Autodesk Inventor part; units mm, degrees
(part 2 of 2)
sketch "Sketch10" plane through (12.7, -57.9553, 48.26) normal (1, 0, 0) x (0, 0, -1)
  line L0 (238.76, 169.0803) -> (-142.24, 169.0803) projected
  circle A0 centre (-74.422, 78.5928) radius 3.175 projected
  circle A1 centre (-74.422, 103.9928) radius 3.175 projected
  circle A2 centre (48.26, 57.9553) radius 3.175 projected
  circle A3 centre (-48.26, 57.9553) radius 3.175 projected
  circle A4 centre (144.78, 57.9553) radius 3.175 projected
  circle A5 centre (-205.74, 124.6303) radius 12.7 projected
  circle A6 centre (302.26, 124.6303) radius 12.7 projected
  line L1 (-205.74, 124.6303) -> (302.26, 124.6303) construction
  line L2 (48.26, 124.6303) -> (48.26, 202.3568) construction
  circle A7 centre (-133.9387, 147.2642) radius 2.413 projected
  circle A8 centre (-131.9736, 159.9642) radius 2.413 projected
  circle A9 centre (230.4587, 147.2642) radius 2.413
  circle A10 centre (228.4936, 159.9642) radius 2.413
  line L3 (238.76, 169.0803) -> (239.9837, 147.2642)
  arc A11 (230.4587, 137.7392) -> (239.9837, 147.2642) centre (230.4587, 147.2642) ccw
  spline S0 degree 4 poles (180.4444, 121.0575) (193.8696, 130.2235) (215.0032, 150.2263) (220.4765, 137.7392) (230.4587, 137.7392) knots 0 0 0 0 0 1 1 1 1 1
  circle A12 centre (81.2991, 80.8647) radius 2.0193 projected
  line L4 (-142.24, 169.0803) -> (-142.24, 124.4818) projected
  arc A13 (-110.574, 77.2765) -> (-142.24, 124.4818) centre (-128.865, 99.2303) ccw projected
  line L5 (-110.574, 77.2765) -> (-54.3105, 46.7892) projected
  arc A14 (-54.3105, 46.7892) -> (-42.2095, 46.7892) centre (-48.26, 57.9553) ccw projected
  line L6 (-42.2095, 46.7892) -> (-7.5631, 65.5629) projected
  arc A15 (7.5631, 65.5629) -> (-7.5631, 65.5629) centre (0, 51.6053) ccw projected
  line L7 (7.5631, 65.5629) -> (42.2095, 46.7892) projected
  arc A16 (42.2095, 46.7892) -> (54.3105, 46.7892) centre (48.26, 57.9553) ccw projected
  line L8 (54.3105, 46.7892) -> (88.9569, 65.5629) projected
  arc A17 (104.0831, 65.5629) -> (88.9569, 65.5629) centre (96.52, 51.6053) ccw projected
  line L9 (104.0831, 65.5629) -> (138.7295, 46.7892) projected
  arc A18 (138.7295, 46.7892) -> (150.8305, 46.7892) centre (144.78, 57.9553) ccw projected
  line L10 (150.8305, 46.7892) -> (207.094, 77.2765) projected
  arc A19 (238.76, 124.4818) -> (207.094, 77.2765) centre (225.385, 99.2303) ccw projected
  line L11 (238.76, 124.4818) -> (238.76, 169.0803) projected
  point P0 (215.721, 140.529)
  dimension "d83" = 254
  constraints: 6 end point, 3 centre point, 2 point on circle, 2 symmetric about line, 1 horizontal, 1 midpoint, 1 vertical, 6 other
  measures "d83" distance from line of L2 L1.start
extrude "Extrusion12" [suppressed]
sketch "Sketch11" plane through (12.7, -57.9553, 48.26) normal (1, 0, 0) x (0, 0, -1)
  circle A0 centre (228.4936, 159.9642) radius 2.413 projected
  circle A1 centre (228.4936, 159.9642) radius 2.413
  point P0 (48.26, 57.9553)
  constraints: 1 centre point, 1 coincident, 1 concentric
extrude "Extrusion13" [suppressed]
sketch "Sketch12" plane through (12.7, -57.9553, 48.26) normal (1, 0, 0) x (0, 0, -1)
  circle A0 centre (224.987, 100.468) radius 6.35 construction
  circle A1 centre (173.2834, 131.5461) radius 6.35 projected
  circle A2 centre (-97.79, 143.6803) radius 7.9375 projected
  circle A3 centre (-47.752, 156.3803) radius 2.0193
  line L0 (238.76, 169.0803) -> (-142.24, 169.0803) projected
  line L1 (44.2912, 144.6069) -> (44.2912, 72.043) projected
  line L2 (97.5225, 158.7615) -> (97.5225, 118.5822) projected
  circle A4 centre (-22.352, 156.3803) radius 2.0193
  circle A5 centre (-47.752, 130.9803) radius 2.0193
  circle A6 centre (-22.352, 130.9803) radius 2.0193
  circle A7 centre (66.04, 105.5803) radius 2.0193
  circle A8 centre (91.44, 105.5803) radius 2.0193
  circle A9 centre (66.04, 80.1803) radius 2.0193
  circle A10 centre (91.44, 80.1803) radius 2.0193
  circle A11 centre (-74.422, 103.9928) radius 3.175 projected
  circle A12 centre (-74.422, 78.5928) radius 3.175 projected
  circle A13 centre (140.335, 92.8803) radius 7.9375 projected
  circle A14 centre (144.78, 57.9553) radius 3.175 projected
  circle A15 centre (230.4587, 147.2642) radius 2.413 projected
  circle A16 centre (176.53, 89.5304) radius 3.175
  circle A17 centre (212.5643, 140.4513) radius 3.175
  circle A18 centre (173.2834, 131.5461) radius 29.845 construction
  circle A19 centre (140.335, 92.8803) radius 23.495 construction
  circle A20 centre (224.987, 100.468) radius 33.02 construction
  line L3 (144.78, 57.9553) -> (176.53, 89.5304) construction
  line L4 (176.53, 89.5304) -> (140.335, 92.8803) construction
  line L5 (176.53, 89.5304) -> (173.2834, 131.5461) construction
  line L6 (176.53, 89.5304) -> (212.5643, 140.4513) construction
  line L7 (212.5643, 140.4513) -> (230.4587, 147.2642) construction
  line L8 (212.5643, 140.4513) -> (173.2834, 131.5461) construction
  circle A21 centre (224.987, 100.468) radius 23.8125 construction
  circle A22 centre (176.53, 89.5304) radius 6.35 construction
  circle A23 centre (212.5643, 140.4513) radius 6.35 construction
  point P0 (48.26, 57.9553)
  dimension "d88" = 12.7
  dimension "d89" = 31.078
  dimension "d90" = 51.7036
  dimension "d94" = 4.0386
  dimension "d97" = 25.4
  dimension "d100" = 25.4
  dimension "d103" = 4.0386
  dimension "d106" = 25.4
  dimension "d109" = 25.4
  dimension "d112" = 50.038
  dimension "d113" = 12.7
  dimension "d114" = 48.895
  dimension "d115" = 12.7
  dimension "d116" = 6.35
  dimension "d117" = 6.35
  dimension "d118" = 59.69
  dimension "d119" = 46.99
  dimension "d120" = 66.04
  dimension "d121" = 47.625
  dimension "d122" = 31.75
  dimension "d124" = 12.7
  dimension "d125" = 12.7
  constraints: 17 centre point, 12 end point, 6 coincident, 2 horizontal, 2 vertical, 12 other
  measures "d88" diameter of A0
  measures "d89" vertical distance of A0.centre A1.centre
  measures "d90" horizontal distance of A0.centre A1.centre
  measures "d94" diameter of A3
  measures "d97" distance of A3.centre A4.centre
  measures "d100" distance of A3.centre A5.centre
  measures "d103" diameter of A7
  measures "d106" distance of A7.centre A8.centre
  measures "d109" distance of A7.centre A9.centre
  measures "d112" horizontal distance of A5.centre A2.centre
  measures "d113" vertical distance of A5.centre A2.centre
  measures "d114" horizontal distance of A13.centre A10.centre
  measures "d115" vertical distance of A13.centre A10.centre
  measures "d116" diameter of A16
  measures "d117" diameter of A17
  measures "d118" diameter of A18
  measures "d119" diameter of A19
  measures "d120" diameter of A20
  measures "d121" diameter of A21
  measures "d122" horizontal distance of L3.end L3.start
  measures "d124" diameter of A22
  measures "d125" diameter of A23
fillet "Fillet4" [suppressed]
fillet "Fillet5" [suppressed]
sketch "Sketch13" plane through (12.7, 0, 0) normal (1, 0, 0) x (0, 0, -1)
  arc A0 (-155.8742, 22.1717) -> (-155.0257, 17.2576) centre (-153.513, 20.0491) ccw projected
  line L0 (-155.0257, 17.2576) -> (-102.5705, -11.1661) projected
  arc A1 (-102.5705, -11.1661) -> (-90.4695, -11.1661) centre (-96.52, 0) ccw projected
  line L1 (-90.4695, -11.1661) -> (-55.8231, 7.6076) projected
  arc A2 (-40.6969, 7.6076) -> (-55.8231, 7.6076) centre (-48.26, -6.35) ccw projected
  line L2 (-40.6969, 7.6076) -> (-6.0505, -11.1661) projected
  arc A3 (-6.0505, -11.1661) -> (6.0505, -11.1661) centre (0, 0) ccw projected
  line L3 (6.0505, -11.1661) -> (40.6969, 7.6076) projected
  arc A4 (55.8231, 7.6076) -> (40.6969, 7.6076) centre (48.26, -6.35) ccw projected
  line L4 (55.8231, 7.6076) -> (90.4695, -11.1661) projected
  arc A5 (90.4695, -11.1661) -> (102.5705, -11.1661) centre (96.52, 0) ccw projected
  line L5 (102.5705, -11.1661) -> (155.0257, 17.2576) projected
  arc A6 (155.0257, 17.2576) -> (155.8742, 22.1717) centre (153.513, 20.0491) ccw projected
  arc A7 (186.305, 68.3353) -> (155.8742, 22.1717) centre (177.125, 41.275) ccw projected
  arc A8 (186.305, 68.3353) -> (190.5, 71.342) centre (187.325, 71.342) ccw projected
  line L6 (190.5, 71.342) -> (190.5, 111.125) projected
  line L7 (190.5, 111.125) -> (-190.5, 111.125) projected
  line L8 (-190.5, 111.125) -> (-190.5, 71.342) projected
  arc A9 (-190.5, 71.342) -> (-186.305, 68.3353) centre (-187.325, 71.342) ccw projected
  arc A10 (-155.8742, 22.1717) -> (-186.305, 68.3353) centre (-177.125, 41.275) ccw projected
  circle A11 centre (-79.2324, 71.4375) radius 3.175 projected
  circle A12 centre (88.2841, 92.075) radius 3.175 projected
  circle A13 centre (182.1987, 89.3089) radius 2.413 projected
  circle A14 centre (-182.1987, 89.3089) radius 2.413 projected
  circle A15 centre (-107.3629, 85.725) radius 11 projected
  circle A16 centre (33.0391, 22.9094) radius 2.0193 projected
  circle A17 centre (-31.9249, 73.9625) radius 2.0193 projected
  circle A18 centre (-31.9249, 99.3625) radius 2.0193 projected
  circle A19 centre (33.0391, 48.3094) radius 2.0193 projected
  circle A20 centre (-57.3249, 99.3625) radius 2.0193 projected
  circle A21 centre (-122.682, 46.0375) radius 3.175 projected
  circle A22 centre (96.52, 0) radius 3.175 projected
  circle A23 centre (0, 0) radius 3.175 projected
  circle A24 centre (-96.52, 0) radius 3.175 projected
  circle A25 centre (-57.3249, 73.9625) radius 2.0193 projected
  circle A26 centre (58.4391, 48.3094) radius 2.0193 projected
  circle A27 centre (58.4391, 22.9094) radius 2.0193 projected
  circle A28 centre (-180.2336, 102.0089) radius 2.413 projected
  circle A29 centre (180.2336, 102.0089) radius 2.413 projected
  circle A30 centre (88.2841, 66.675) radius 3.175 projected
  circle A31 centre (-79.2324, 103.1875) radius 3.175 projected
  circle A32 centre (132.7341, 17.4625) radius 3.175 projected
  circle A33 centre (-147.5038, 79.375) radius 14.2875 projected
  circle A34 centre (-122.682, 20.6375) radius 3.175 projected
  line L9 (-187.325, 107.95) -> (187.325, 107.95)
  line L10 (187.325, 107.95) -> (187.325, 71.342)
  arc A35 (187.325, 71.342) -> (153.513, 20.0491) centre (177.125, 41.275) ccw
  line L11 (153.513, 20.0491) -> (101.0579, -8.3746)
  arc A36 (91.9821, -8.3746) -> (101.0579, -8.3746) centre (96.52, 0) ccw
  line L12 (91.9821, -8.3746) -> (57.3358, 10.3991)
  arc A37 (57.3358, 10.3991) -> (39.1842, 10.3991) centre (48.26, -6.35) ccw
  line L13 (39.1842, 10.3991) -> (4.5379, -8.3746)
  arc A38 (-4.5379, -8.3746) -> (4.5379, -8.3746) centre (0, 0) ccw
  line L14 (-4.5379, -8.3746) -> (-39.1842, 10.3991)
  arc A39 (-39.1842, 10.3991) -> (-57.3358, 10.3991) centre (-48.26, -6.35) ccw
  line L15 (-57.3358, 10.3991) -> (-91.9821, -8.3746)
  arc A40 (-101.0579, -8.3746) -> (-91.9821, -8.3746) centre (-96.52, 0) ccw
  line L16 (-101.0579, -8.3746) -> (-153.513, 20.0491)
  arc A41 (-153.513, 20.0491) -> (-187.325, 71.342) centre (-177.125, 41.275) ccw
  line L17 (-187.325, 71.342) -> (-187.325, 107.95)
  circle A42 centre (-147.5038, 79.375) radius 17.4625
  circle A43 centre (-107.3629, 85.725) radius 14.175
  circle A44 centre (-79.2324, 103.1875) radius 6.35
  circle A45 centre (-122.682, 46.0375) radius 6.35
  circle A46 centre (-122.682, 20.6375) radius 6.35
  circle A47 centre (-79.2324, 71.4375) radius 6.35
  circle A48 centre (88.2841, 66.675) radius 6.35
  circle A49 centre (88.2841, 92.075) radius 6.35
  circle A50 centre (132.7341, 17.4625) radius 6.35
  circle A51 centre (-57.3249, 99.3625) radius 5.1943
  circle A52 centre (-31.9249, 99.3625) radius 5.1943
  circle A53 centre (-57.3249, 73.9625) radius 5.1943
  circle A54 centre (-31.9249, 73.9625) radius 5.1943
  circle A55 centre (33.0391, 48.3094) radius 5.1943
  circle A56 centre (58.4391, 48.3094) radius 5.1943
  circle A57 centre (33.0391, 22.9094) radius 5.1943
  circle A58 centre (58.4391, 22.9094) radius 5.1943
  circle A59 centre (180.2336, 102.0089) radius 5.588
  circle A60 centre (182.1987, 89.3089) radius 5.588
  circle A61 centre (96.52, 0) radius 6.35
  circle A62 centre (0, 0) radius 6.35
  circle A63 centre (-96.52, 0) radius 6.35
  line L18 (-147.5038, 79.375) -> (-107.3629, 85.725) construction
  line L19 (-107.3629, 85.725) -> (-79.2324, 103.1875) construction
  line L20 (-79.2324, 103.1875) -> (-57.3249, 99.3625) construction
  line L21 (-57.3249, 99.3625) -> (-31.9249, 99.3625) construction
  line L22 (-31.9249, 99.3625) -> (88.2841, 92.075) construction
  line L23 (88.2841, 92.075) -> (135.2431, 65.2528) construction
  line L24 (108.4771, 34.6719) -> (132.7341, 17.4625) construction
  line L25 (132.7341, 17.4625) -> (96.52, 0) construction
  line L26 (96.52, 0) -> (58.4391, 22.9094) construction
  line L27 (58.4391, 22.9094) -> (33.0391, 48.3094) construction
  line L28 (33.0391, 48.3094) -> (-31.9249, 73.9625) construction
  line L29 (-31.9249, 73.9625) -> (-57.3249, 99.3625) construction
  line L30 (-147.5038, 79.375) -> (-122.682, 46.0375) construction
  line L31 (-122.682, 46.0375) -> (-122.682, 20.6375) construction
  line L32 (-122.682, 20.6375) -> (-96.52, 0) construction
  line L33 (-96.52, 0) -> (-79.2324, 71.4375) construction
  line L34 (-79.2324, 71.4375) -> (-57.3249, 73.9625) construction
  line L35 (-57.3249, 73.9625) -> (-31.9249, 73.9625) construction
  line L36 (-31.9249, 73.9625) -> (0, 0) construction
  line L37 (0, 0) -> (33.0391, 22.9094) construction
  line L38 (33.0391, 22.9094) -> (33.0391, 48.3094) construction
  line L39 (-107.3629, 85.725) -> (-79.2324, 71.4375) construction
  line L40 (-31.9249, 99.3625) -> (-31.9249, 73.9625) construction
  line L41 (-57.3249, 99.3625) -> (-57.3249, 73.9625) construction
  line L42 (33.0391, 48.3094) -> (58.4391, 48.3094) construction
  line L43 (58.4391, 48.3094) -> (58.4391, 22.9094) construction
  line L44 (33.0391, 22.9094) -> (58.4391, 22.9094) construction
  line L45 (108.4771, 34.6719) -> (58.4391, 22.9094) construction
  line L46 (108.4771, 34.6719) -> (58.4391, 48.3094) construction
  line L47 (108.4771, 34.6719) -> (88.2841, 66.675) construction
  line L48 (88.2841, 66.675) -> (135.2431, 65.2528) construction
  line L49 (88.2841, 66.675) -> (88.2841, 92.075) construction
  line L50 (108.4771, 34.6719) -> (135.2431, 65.2528) construction
  line L51 (135.2431, 65.2528) -> (182.1987, 89.3089) construction
  line L52 (135.2431, 65.2528) -> (180.2336, 102.0089) construction
  line L53 (88.2841, 92.075) -> (180.2336, 102.0089) construction
  line L54 (-180.2336, 102.0089) -> (-147.5038, 79.375) construction
  line L55 (-182.1987, 89.3089) -> (-147.5038, 79.375) construction
  circle A64 centre (135.2431, 65.2528) radius 14.2875 projected
  circle A65 centre (135.2431, 65.2528) radius 17.4625
  circle A66 centre (-180.2336, 102.0089) radius 5.588
  circle A67 centre (-182.1987, 89.3089) radius 5.588
  circle A68 centre (108.4771, 34.6719) radius 11 projected
  line L56 (132.7341, 17.4625) -> (135.2431, 65.2528) construction
  line L57 (58.4391, 48.3094) -> (88.2841, 66.675) construction
  line L58 (58.4391, 48.3094) -> (88.2841, 92.075) construction
  line L59 (33.0391, 48.3094) -> (-31.9249, 99.3625) construction
  line L60 (33.0391, 48.3094) -> (36.2167, 95.2315) construction
  line L61 (58.4391, 48.3094) -> (36.2167, 95.2315) construction
  line L62 (-57.3249, 73.9625) -> (-48.26, 12.7) construction
  line L63 (-122.682, 46.0375) -> (-79.2324, 71.4375) construction
  dimension "d300" = 3.175
  dimension "d301" = 3.175
  dimension "d302" = 3.175
  dimension "d303" = 3.175
  dimension "d304" = 3.175
  dimension "d307" = 3.175
  dimension "d308" = 3.175
  dimension "d309" = 3.175
  constraints: 110 end point, 32 centre point, 17 equal radius, 15 point on circle, 3 perpendicular, 2 coincident, 2 horizontal, 2 parallel, 1 point on line, 1 vertical, 15 other
  measures "d300" distance between parallel lines of L7 L9
  measures "d301" radial gap between concentric circles of A33 A42
  measures "d302" radial gap between concentric circles of A15 A43
  measures "d303" radial gap between concentric circles of A31 A44
  measures "d304" radial gap between concentric circles of A20 A51
  measures "d307" radial gap between concentric circles of A29 A59
  measures "d308" radial gap between concentric circles of A13 A60
  measures "d309" radial gap between concentric circles of A22 A61
sketch "Sketch14" plane through (12.7, 0, 0) normal (1, 0, 0) x (0, 0, -1)
  circle A0 centre (-147.5038, 79.375) radius 14.2875 projected
  circle A1 centre (-107.3629, 85.725) radius 11 projected
  circle A2 centre (108.4771, 34.6719) radius 11 projected
  circle A3 centre (135.2431, 65.2528) radius 14.2875 projected
  circle A4 centre (-147.5038, 79.375) radius 6.35
  circle A5 centre (-107.3629, 85.725) radius 6.35
  circle A6 centre (108.4771, 34.6719) radius 6.35
  circle A7 centre (135.2431, 65.2528) radius 6.35
  point P0 (0, 0)
  dimension "d327" = 12.7
  dimension "d328" = 12.7
  dimension "d329" = 12.7
  dimension "d330" = 12.7
  constraints: 4 centre point, 4 coincident
  measures "d327" diameter of A4
  measures "d328" diameter of A5
  measures "d329" diameter of A6
  measures "d330" diameter of A7
extrude "Extrusion14" [suppressed]
extrude "Extrusion15" [suppressed]
sketch "Sketch17" plane through (0, 0, 0) normal (1, 0, 0) x (0, 1, 0)
  circle A0 centre (80.3177, 148.0067) radius 2.54
  circle A1 centre (41.275, 177.125) radius 2.54
  circle A2 centre (46.0375, 122.682) radius 3.175 projected
  circle A3 centre (20.6375, 122.682) radius 3.175 projected
  circle A4 centre (80.3177, 148.0067) radius 7.62
  circle A5 centre (41.275, 177.125) radius 7.62
  line L0 (34.1796, 179.9035) -> (12.9508, 125.692)
  line L1 (45.8306, 183.2333) -> (84.8733, 154.115)
  line L2 (51.041, 116.1162) -> (84.9363, 141.946)
  line L3 (20.6375, 114.427) -> (46.0375, 114.427)
  circle A6 centre (46.0375, 122.682) radius 8.255
  circle A7 centre (20.6375, 122.682) radius 8.255
  point P0 (0, 0)
  dimension "d349" = 5.08
  dimension "d350" = 5.08
  dimension "d351" = 5.08
  dimension "d352" = 5.08
  dimension "d356" = 5.08
  dimension "d357" = 5.08
  constraints: 8 end point, 4 centre point, 4 point on circle, 4 tangent, 2 horizontal, 1 coincident, 8 other
  measures "d349" diameter of A0
  measures "d350" diameter of A1
  measures "d351" radial gap between concentric circles of A0 A4
  measures "d352" radial gap between concentric circles of A1 A5
extrude "Extrusion17" add sketch "Sketch17" along normal blind 1.5875
body "Solid1"
